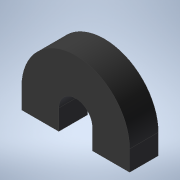
# Autodesk Inventor part: Riemenscheibe_Adjustment_Disk
Saved by Autodesk Inventor 2022 (Build 260153000, 153)
## iProperties
Created: 2023-08-01
Part Number: Riemenscheibe_Adjustment_Disk
Material: Generisch
Document SubType Name: Modeling
Designer: aewalder
Density: 1 g/cm^3
Appearance: Vorgabe
Author: aewalder
Autodesk Inventor part; units mm, degrees
ref_plane "YZ Plane" through (0, 0, 0) normal (1, 0, 0) x (0, 1, 0)
ref_plane "XZ Plane" through (0, 0, 0) normal (0, 1, 0) x (-1, 0, 0)
ref_plane "XY Plane" through (0, 0, 0) normal (0, 0, 1) x (1, 0, 0)
sketch "Sketch1" plane through (0, 0, 0) normal (0, 0, 1) x (1, 0, 0)
  circle A0 centre (0, 0) radius 2.5
  circle A1 centre (0, 0) radius 8
  line L0 (-8, 0) -> (8, 0)
  point P0 (-2.5, 0)
  point P1 (2.5, 0)
  dimension "d0" = 16
  dimension "d1" = 5
  constraints: 2 centre point, 2 coincident, 2 end point, 2 point on circle, 1 horizontal, 1 midpoint
  measures "d0" diameter of A1
  measures "d1" diameter of A0
extrude "Extrusion1" add sketch "Sketch1" along normal blind 4.25 contours A0 L0 A1 picked at (-6.065, 0.8376)
sketch "Sketch2" plane through (-8, 0, 0) normal (0, -1, 0) x (1, 0, 0)
  line L0 (0, 0) -> (5.5, 0) projected
  line L1 (5.5, 0) -> (5.5, 4.25) projected
  line L2 (0, 4.25) -> (5.5, 4.25) projected
  line L3 (0, 0) -> (0, 4.25) projected
  line L4 (10.5, 0) -> (16, 0) projected
  line L5 (16, 0) -> (16, 4.25) projected
  line L6 (10.5, 4.25) -> (16, 4.25) projected
  line L7 (10.5, 0) -> (10.5, 4.25) projected
  point P0 (8, 0)
extrude "Extrusion2" add sketch "Sketch2" along normal blind 3
body "Solid1"
